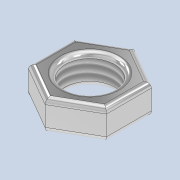
# Autodesk Inventor part: M5 Nut Silver
Saved by Autodesk Inventor 2022 (Build 260153000, 153)
## iProperties
Created: 2021-07-18
Part Number: M5 Nut Silver
Material: Generic
Document SubType Name: Modeling
Designer: Coy
Density: 1 g/cm^3
Appearance: Chrome - Polished
Author: Coy
Autodesk Inventor part; units mm, degrees
ref_plane "YZ Plane" through (0, 0, 0) normal (1, 0, 0) x (0, 1, 0)
ref_plane "XZ Plane" through (0, 0, 0) normal (0, 1, 0) x (-1, 0, 0)
ref_plane "XY Plane" through (0, 0, 0) normal (0, 0, 1) x (1, 0, 0)
sketch "Sketch1" plane through (0, 0, 0) normal (0, 1, 0) x (-1, 0, 0)
  line L0 (3.95, -2.2805) -> (0, -4.5611)
  line L1 (0, -4.5611) -> (-3.95, -2.2805)
  line L2 (-3.95, -2.2805) -> (-3.95, 2.2805)
  line L3 (-3.95, 2.2805) -> (0, 4.5611)
  line L4 (0, 4.5611) -> (3.95, 2.2805)
  line L5 (3.95, 2.2805) -> (3.95, -2.2805)
  circle A0 centre (0, 0) radius 2.5
  dimension "d0" = 3.95
  dimension "d1" = 5
  constraints: 12 end point, 2 coincident, 1 centre point, 13 other
  measures "d0" distance from line of point (0, 0) L5
  measures "d1" diameter of A0
extrude "Extrusion1" add sketch "Sketch1" along normal blind 3
fillet "Fillet1" radius 0.5 14 edges at (3.95, 3, 0) (1.975, 3, -3.4208) (-1.975, 3, -3.4208) (-3.95, 3, 0) (-1.975, 3, 3.4208) (1.975, 3, 3.4208) (3.95, 0, 0) (1.975, 0, 3.4208) (-1.975, 0, 3.4208) (-3.95, 0, 0) (-1.975, 0, -3.4208) (1.975, 0, -3.4208) (2.5, 0, 0) (2.5, 3, 0)
thread "Thread1" size "M5x0.8" class "6H" standard "ANSI Metric M Profile" full length
body "Solid1"
